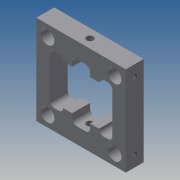
# Autodesk Inventor part: Holder
Saved by Autodesk Inventor 2015 (Build 190159000, 159)
## iProperties
Created: 2014-07-11
Part Number: Holder
Material: Generic
Document SubType Name: Modeling
Designer: jad211
Density: 1 g/cm^3
Appearance: Default
Author: jad211
Autodesk Inventor part; units mm, degrees
ref_plane "YZ Plane" through (0, 0, 0) normal (1, 0, 0) x (0, 1, 0)
ref_plane "XZ Plane" through (0, 0, 0) normal (0, 1, 0) x (-1, 0, 0)
ref_plane "XY Plane" through (0, 0, 0) normal (0, 0, 1) x (1, 0, 0)
sketch "Sketch1" plane through (0, 0, 0) normal (0, 1, 0) x (-1, 0, 0)
  line L0 (20, 20) -> (20, -20)
  line L1 (20, -20) -> (-20, -20)
  line L2 (-20, -20) -> (-20, 20)
  line L3 (-20, 20) -> (20, 20)
  line L4 (-15, 15) -> (-15, -15) construction
  line L5 (-15, -15) -> (15, -15) construction
  line L6 (15, -15) -> (15, 15) construction
  line L7 (15, 15) -> (-15, 15) construction
  circle A0 centre (15, 15) radius 3.05
  circle A1 centre (15, -15) radius 3.05
  circle A2 centre (-15, -15) radius 3.05
  circle A3 centre (-15, 15) radius 3.05
  line L8 (0, 0) -> (-18.5703, 0) construction
  line L9 (-8, 9) -> (-8, 9)
  line L10 (-10, 11) -> (-12, 11)
  line L11 (-14, 9) -> (-14, -9)
  line L12 (-12, -11) -> (-10, -11)
  line L13 (-8, -9) -> (-8, -9)
  line L14 (8, -9) -> (8, -9)
  line L15 (10, -11) -> (12, -11)
  line L16 (14, -9) -> (14, 9)
  line L17 (12, 11) -> (10, 11)
  line L18 (8, 9) -> (8, 9)
  line L19 (0, 0) -> (0, 18.05) construction
  line L20 (0, 0) -> (-18.05, 0) construction
  arc A4 (-12, 11) -> (-14, 9) centre (-12, 9) ccw
  arc A5 (-8, 9) -> (-10, 11) centre (-10, 9) ccw
  arc A6 (-10, -11) -> (-8, -9) centre (-10, -9) ccw
  arc A7 (-14, -9) -> (-12, -11) centre (-12, -9) ccw
  arc A8 (8, -9) -> (10, -11) centre (10, -9) ccw
  arc A9 (12, -11) -> (14, -9) centre (12, -9) ccw
  arc A10 (14, 9) -> (12, 11) centre (12, 9) ccw
  arc A11 (10, 11) -> (8, 9) centre (10, 9) ccw
  line L21 (8, 9) -> (4, 9)
  line L22 (4, 9) -> (4, 11)
  line L23 (2, 13) -> (-2, 13)
  line L24 (-4, 11) -> (-4, 9)
  line L25 (-4, 9) -> (-8, 9)
  line L26 (-8, -9) -> (-4, -9)
  line L27 (-4, -9) -> (-4, -11)
  line L28 (-2, -13) -> (2, -13)
  line L29 (4, -11) -> (4, -9)
  line L30 (8, -9) -> (4, -9)
  arc A12 (4, 11) -> (2, 13) centre (2, 11) ccw
  arc A13 (-2, 13) -> (-4, 11) centre (-2, 11) ccw
  arc A14 (2, -13) -> (4, -11) centre (2, -11) ccw
  arc A15 (-4, -11) -> (-2, -13) centre (-2, -11) ccw
  point P0 (-8, 11)
  point P1 (-14, 11)
  point P2 (-8, -11)
  point P3 (8, -11)
  point P4 (14, -11)
  point P5 (8, 11)
  point P6 (-4, 13)
  point P7 (-4, -13)
  point P8 (4, -13)
  dimension "d0" = 40
  dimension "d1" = 40
  dimension "d2" = 30
  dimension "d3" = 6.1
  dimension "d53" = 20
  dimension "d54" = 15
  dimension "d57" = 8
  dimension "d58" = 16
  dimension "d59" = 22
  dimension "d60" = 6
  dimension "d61" = 2
  dimension "d96" = 4
  dimension "d97" = 8
  dimension "d98" = 4
  dimension "d99" = 2
  constraints: 62 end point, 29 point on line, 24 point on circle, 24 tangent, 16 centre point, 13 equal radius, 6 perpendicular, 4 coincident, 4 horizontal, 1 collinear, 4 other
  measures "d0" distance of L0.end L1.end
  measures "d1" distance of L0.start L0.end
  measures "d2" distance of L5.end L6.end
  measures "d3" diameter of A0
  measures "d53" distance from line of L8.start L1
  measures "d54" horizontal distance of L8.start L4.start
  measures "d57" horizontal distance of L13.end L8.start
  measures "d58" distance of L13.end L14.start
  measures "d59" distance between parallel lines of L12 L10
  measures "d60" distance of point (-8, 11) point (-14, 11)
  measures "d61" radius of A4
  measures "d96" distance of point (-4, 13) L24.end
  measures "d97" distance of L24.end L21.end
  measures "d98" distance of L26.end point (-4, -13)
  measures "d99" radius of A12
extrude "Extrusion5" add sketch "Sketch1" along normal blind 8
sketch "Sketch8" plane through (20, 0, -20) normal (0, 0, -1) x (-1, 0, 0)
  circle A0 centre (20, 4) radius 1.5
  point P0 (20, 0)
  dimension "d100" = 4
  dimension "d101" = 3
  constraints: 1 centre point
  measures "d100" distance of point (20, 0) A0.centre
  measures "d101" diameter of A0
sketch "Sketch9" plane through (20, 0, 20) normal (1, 0, 0) x (0, 0, -1)
  line L0 (40, 0) -> (0, 0) projected
  line L1 (40, 0) -> (40, 8) projected
  line L2 (0, 8) -> (40, 8) projected
  line L3 (0, 0) -> (0, 8) projected
  point P0 (20, 0)
  point P1 (5, 4)
  point P2 (35, 4)
  dimension "d104" = 5
  dimension "d105" = 5
  dimension "d106" = 4
  dimension "d107" = 4
  measures "d104" distance from line of L3 point (5, 4)
  measures "d105" distance from line of L1 point (35, 4)
  measures "d106" distance from line of L0 point (5, 4)
  measures "d107" distance from line of L0 point (35, 4)
hole "Hole1" at (20, 4, 15) at (20, 4, -15) direction (-1, 0, 0) diameter 2.013 depth 5 tip angle 118 thread size "M2.5x0.45" class "6H" standard "ISO Metric profile"
sketch "Sketch10" plane through (-20, 0, -20) normal (-1, 0, 0) x (0, 0, 1)
  circle A0 centre (35, 4) radius 1.0065 projected
  circle A1 centre (5, 4) radius 1.0065 projected
  point P0 (20, 0)
  point P1 (33.9935, 4)
  point P2 (3.9935, 4)
  constraints: 2 coincident, 2 horizontal alignment, 2 other
hole "Hole2" at (-20, 4, 15) at (-20, 4, -15) direction (1, 0, 0) diameter 2.013 depth 5 tip angle 118 thread size "M2.5x0.45" class "6H" standard "ISO Metric profile"
hole "Hole3" at (0, 4, -20) direction (0, 0, 1) diameter 3.1 end through all
equation "\"d1\" = d0"
body "Solid2"
